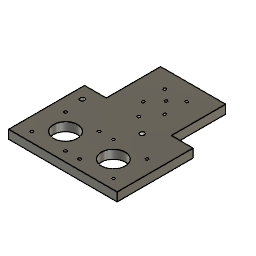
XY Plotter Central Plate (Autodesk Fusion 360 design; units mm, degrees)
Autodesk Fusion 360 part; units mm, degrees
sketch "Sketch1" plane through (0, 0, 0) normal (0, 0, 1) x (1, 0, 0)
  line L0 (50, 35) -> (-50, 35)
  line L1 (-50, 35) -> (-50, -35)
  line L2 (-50, -35) -> (50, -35)
  line L3 (50, -35) -> (50, 35)
  line L4 (50, 35) -> (-50, -35) construction
  line L5 (-50, 35) -> (50, -35) construction
  line L6 (-30, 35) -> (-30, 85)
  line L7 (-30, 85) -> (30, 85)
  line L8 (30, 85) -> (30, 35)
  circle A0 centre (-22, -10.5) radius 11
  circle A1 centre (22, -10.5) radius 11
  point P0 (-37.5, -26)
  point P1 (-6.5, -26)
  point P2 (-37.5, 5)
  point P3 (-6.5, 5)
  point P4 (6.5, -26)
  point P5 (37.5, -26)
  point P6 (6.5, 5)
  point P7 (37.5, 5)
  point P8 (-40, 23)
  point P9 (15, 23)
  point P10 (10, 48.9294)
  point P11 (10, 68.9294)
  point P12 (-10, 68.9294)
  point P13 (-10, 48.9294)
  point P14 (0, 35)
  point P15 (0, 60)
  dimension "d1" = 100
  dimension "d2" = 70
  dimension "d3" = 9
  dimension "d6" = 31
  dimension "d7" = 31
  dimension "d8" = 12.5
  dimension "d10" = 31
  dimension "d13" = 12.5
  dimension "d15" = 12
  dimension "d16" = 10
  dimension "d17" = 55
  dimension "d18" = 50
  dimension "d19" = 60
  dimension "d20" = 20
  dimension "d21" = 20
  dimension "d22" = 20
  dimension "d23" = 20
  dimension "d37" = 22
  dimension "d38" = 15.5
  dimension "d39" = 15.5
  dimension "d40" = 22
  dimension "d41" = 15.5
  dimension "d42" = 21.9203
  dimension "d45" = 25
  constraint horizontal L0
  constraint perpendicular L0 L1
  constraint parallel L0 L2
  constraint parallel L1 L3
  constraint coincident L4 origin
  constraint coincident L5 origin
  constraint coincident L0 L6.start
  constraint perpendicular L0 L6
  constraint perpendicular L6 L7
  constraint coincident L0 L8.end
  constraint perpendicular L0 L8
  constraint midpoint L0 P14
  measures "d1" distance of L1.end L2.end
  measures "d2" distance of L0.end L1.end
  measures "d3" distance of L2 P0
  measures "d6" distance of P0 P1
  measures "d7" distance of P0 P2
  measures "d8" distance of L1 P0
  measures "d10" distance of P4 P5
  measures "d13" distance of L3 P5
  measures "d15" distance of L0 P8
  measures "d16" distance of L1 P8
  measures "d17" distance of P8 P9
  measures "d18" distance of L6.start L6.end
  measures "d19" distance of L6.end L7.end
  measures "d20" distance of L1 L6
  measures "d21" distance of L8 P11
  measures "d22" distance of P10 P11
  measures "d23" distance of P11 P12
  measures "d37" diameter of A0
  measures "d38" vertical distance of P0 A0.centre
  measures "d39" horizontal distance of P2 A0.centre
  measures "d40" diameter of A1
  measures "d41" vertical distance of P5 A1.centre
  measures "d42" distance of P4 A1.centre
  measures "d45" distance of P14 P15
extrude "Extrude1" add sketch "Sketch1" against normal blind 8 contours L0 L1 L2 L3 | L0 L6 L7 L8 | A0 | A1
hole "Hole1" at (-37.5, 5, 0) at (-37.5, -26, 0) at (-6.5, -26, 0) at (6.5, -26, 0) at (-6.5, 5, 0) at (6.5, 5, 0) at (37.5, 5, 0) at (37.5, -26, 0) at (-10, 48.9294, 0) at (-10, 68.9294, 0) at (0, 60, 0) at (10, 68.9294, 0) at (0, 35, 0) at (10, 48.9294, 0) direction (0, 0, -1) diameter 2.529 depth 40 tip angle 118
thread "Thread1" "ISO Metric profile 3.0 M3x0.5 M3x0.5 6H" thread offset 0 thread depth 7.4
hole "Hole2" at (15, 23, 0) at (-40, 23, 0) direction (0, 0, -1) diameter 4.234 depth 20 tip angle 118
thread "Thread2" "ISO Metric profile 5.0 M5x0.8 M5x0.8 6H" thread offset 0 thread depth 7.4
extrude "Extrude2" cut sketch "Sketch1" against normal blind 20 contours A0 | A1
equation "d38 = ( 31 / 2 ) * 1 mm"
equation "d39 = ( 31 / 2 ) * 1 mm"
equation "d41 = ( 31 / 2 ) * 1 mm"
equation "d42 = ( 31 / 2 * sqrt(2) ) * 1 mm"
